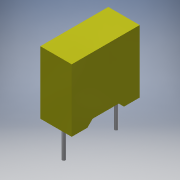
# Autodesk Inventor part: CAP-SUP
Saved by Autodesk Inventor 2018.3 (Build 223284000, 284)
## iProperties
Created: 2021-04-20
Part Number: CAP-SUP
Material: Genérico
Document SubType Name: Modeling
Designer: laguerre
Density: 8.47 g/cm^3
Appearance: Amarillo
Author: laguerre
Autodesk Inventor part; units mm, degrees
ref_plane "YZ Plane" through (0, 0, 0) normal (1, 0, 0) x (0, 1, 0)
ref_plane "XZ Plane" through (0, 0, 0) normal (0, 1, 0) x (-1, 0, 0)
ref_plane "XY Plane" through (0, 0, 0) normal (0, 0, 1) x (1, 0, 0)
sketch "Boceto39" plane through (0, 0, 0) normal (0, 0, 1) x (1, 0, 0)
  line L0 (-6.5, 12) -> (6.5, 12)
  line L1 (6.5, 12) -> (6.5, 0)
  line L2 (-6.5, 0) -> (-6.5, 12)
  line L3 (-5, 0) -> (-5, -4.6401) construction
  line L4 (5, 0) -> (5, -3.6883) construction
  line L5 (-3.5, 0) -> (-2.5, 1)
  line L6 (-2.5, 1) -> (2.5, 1)
  line L7 (2.5, 1) -> (3.5, 0)
  line L8 (6.5, 0) -> (3.5, 0)
  line L9 (-3.5, 0) -> (-6.5, 0)
  point P0 (0, 0)
  point P1 (0, 0)
  point P2 (0, 1)
  point P3 (0, 12)
  point P4 (-5, 0)
  dimension "d373" = 13
  dimension "d374" = 12
  dimension "d375" = 10
  dimension "d376" = 5
  dimension "d379" = 5
  dimension "d380" = 45
  dimension "d381" = 1
  constraints: 20 end point, 5 midpoint, 3 parallel, 2 horizontal, 2 perpendicular, 2 vertical, 2 vertical alignment, 1 coincident, 1 collinear, 1 horizontal alignment
  measures "d373" distance of L0.start L0.end
  measures "d374" distance of L2.start L0.start
  measures "d375" distance between parallel lines of L3 L4
  measures "d376" distance from line of point (0, 0) L3
  measures "d379" distance of L5.end L6.end
  measures "d380" angle of L7 L8
  measures "d381" distance between parallel lines of L9 L6
extrude "Extrusión13" add sketch "Boceto39" along normal mid plane 6
sketch "Boceto40" plane through (3.5, 0, 3) normal (0, -1, 0) x (1, 0, 0)
  line L0 (3, 0) -> (3, -6) projected
  line L1 (0, 0) -> (3, 0) projected
  line L2 (0, 0) -> (0, -6) projected
  line L3 (3, -6) -> (0, -6) projected
  line L4 (-7, 0) -> (-7, -6) projected
  line L5 (-10, 0) -> (-7, 0) projected
  line L6 (-10, 0) -> (-10, -6) projected
  line L7 (-7, -6) -> (-10, -6) projected
  circle A0 centre (1.5, -3) radius 0.3
  circle A1 centre (-8.5, -3) radius 0.3
  point P0 (-3.5, -3)
  dimension "d384" = 0.6
  dimension "d385" = 10
  dimension "d386" = 5
  constraints: 2 centre point, 2 horizontal alignment, 1 equal radius
  measures "d384" diameter of A1
  measures "d385" distance of A1.centre A0.centre
  measures "d386" distance of point (-3.5, -3) A0.centre
extrude "Extrusión14" add sketch "Boceto40" along normal blind 6 contours A0 | A1
